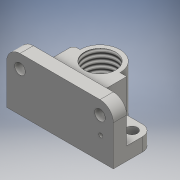
# Autodesk Inventor part: Part1
Saved by Autodesk Inventor 2016 (Build 200138000, 138)
## iProperties
Created: 2018-10-25
Part Number: Part1
Material: Generic
Document SubType Name: Modeling
Designer: dqm_r
Density: 1 g/cm^3
Appearance: Default
Author: dqm_r
Autodesk Inventor part; units mm, degrees
ref_plane "YZ Plane" through (0, 0, 0) normal (1, 0, 0) x (0, 1, 0)
ref_plane "XZ Plane" through (0, 0, 0) normal (0, 1, 0) x (-1, 0, 0)
ref_plane "XY Plane" through (0, 0, 0) normal (0, 0, 1) x (1, 0, 0)
sketch "Sketch1" plane through (0, 0, 0) normal (0, 1, 0) x (-1, 0, 0)
  line L0 (40, 10) -> (40, -20)
  line L1 (40, -20) -> (-40, -20)
  line L2 (-40, -20) -> (-40, 10)
  line L3 (-30, 20) -> (30, 20)
  line L4 (40, 20) -> (-40, -20) construction
  line L5 (40, -20) -> (-40, 20) construction
  arc A0 (40, 10) -> (30, 20) centre (30, 10) ccw
  arc A1 (-30, 20) -> (-40, 10) centre (-30, 10) ccw
  circle A2 centre (30, 10) radius 4
  circle A3 centre (-30, 10) radius 4
  point P0 (0, 0)
  dimension "d0" = 40
  dimension "d1" = 80
  dimension "d2" = 20
  dimension "d3" = 20
  dimension "d4" = 8
  dimension "d5" = 8
  constraints: 12 end point, 4 centre point, 4 point on circle, 4 tangent, 2 coincident, 2 midpoint, 2 parallel, 1 perpendicular, 1 vertical
  measures "d0" distance of L4.start L0.end
  measures "d1" distance of L0.end L1.end
  measures "d2" diameter of A0
  measures "d3" diameter of A1
  measures "d4" diameter of A2
  measures "d5" diameter of A3
extrude "Extrusion1" add sketch "Sketch1" along normal blind 10
sketch "Sketch2" plane through (40, 0, -20) normal (0, 0, -1) x (-1, 0, 0)
  line L0 (70, 10) -> (10, 10) projected
  line L1 (40, 10) -> (60, 10)
  line L2 (40, 10) -> (20, 10)
  line L3 (60, 10) -> (60, 30)
  line L4 (60, 30) -> (20, 30)
  line L5 (20, 30) -> (20, 10)
  point P0 (40, 0)
  dimension "d8" = 20
  dimension "d9" = 20
  dimension "d10" = 20
  constraints: 10 end point, 3 perpendicular, 2 point on line, 1 midpoint
  measures "d8" distance of L1.start L1.end
  measures "d9" distance of L1.start L2.end
  measures "d10" distance of L1.end L3.end
extrude "Extrusion2" add sketch "Sketch2" against normal blind 35
sketch "Sketch3" plane through (40, 0, 15) normal (0, 0, 1) x (1, 0, 0)
  line L0 (-20, 30) -> (-60, 30) projected
  circle A0 centre (-40, 30) radius 15
  point P0 (-40, 0)
  dimension "d13" = 30
  constraints: 1 centre point, 1 midpoint
  measures "d13" diameter of A0
extrude "Extrusion3" cut sketch "Sketch3" against normal blind 35
sketch "Sketch4" plane through (40, 0, -20) normal (0, 0, -1) x (-1, 0, 0)
  line L0 (20, 10) -> (20, 30) projected
  line L1 (20, 30) -> (8.1955, 30)
  circle A0 centre (8, 22) radius 4
  line L2 (0, 10) -> (20, 10) projected
  line L3 (0, 10) -> (20, 10)
  line L4 (20, 10) -> (20, 30)
  line L5 (0, 10) -> (0, 22)
  line L6 (8, 30) -> (8.1955, 30)
  arc A1 (8, 30) -> (0, 22) centre (8, 22) ccw
  point P0 (40, 0)
  dimension "d17" = 8
  dimension "d18" = 16
  constraints: 10 end point, 2 centre point, 2 point on circle, 2 tangent, 1 coincident, 1 collinear, 1 horizontal, 1 perpendicular, 1 vertical
  measures "d17" diameter of A0
  measures "d18" diameter of A1
extrude "Extrusion4" add sketch "Sketch4" against normal blind 10
mirror "Mirror1" about plane through (0, 0, 0) normal (1, 0, 0) of "Extrusion4"
chamfer "Chamfer1" distance 2 angle 45 1 edges at (-20, 30, 2.5)
sketch "Sketch5" plane through (40, 0, 15) normal (0, 0, 1) x (1, 0, 0)
  circle A0 centre (-40, 30) radius 15
  point P0 (-40, 0)
  point P1 (-25, 30)
  constraints: 1 centre point
extrude "Extrusion5" add sketch "Sketch5" against normal up to surface (35 mm away)
sketch "Sketch6" plane through (40, 0, 15) normal (0, 0, 1) x (1, 0, 0)
  arc A0 (-25, 30) -> (-55, 30) centre (-40, 30) ccw projected
  circle A1 centre (-40, 30) radius 11.7834
  point P0 (-40, 0)
  constraints: 1 centre point, 1 coincident
extrude "Extrusion6" cut sketch "Sketch6" against normal through all
thread "Thread1" size "M30x3.5" class "6H" standard "ANSI Metric M Profile" full length
hole "Hole1" at (30.6261, 10, -2.8857) direction (0, -1, 0) diameter 3 end through all countersink diameter 7 countersink angle 90
body "Solid1"
